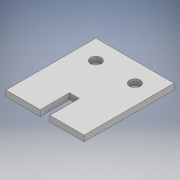
# Autodesk Inventor part: Camera_Mount
Saved by Autodesk Inventor 2017 (Build 210142000, 142)
## iProperties
Created: 2017-01-29
Part Number: Camera_Mount
Material: Generic
Document SubType Name: Modeling
Designer: willt
Density: 1 g/cm^3
Appearance: Default
Author: willt
Autodesk Inventor part; units mm, degrees
ref_plane "YZ Plane" through (0, 0, 0) normal (1, 0, 0) x (0, 1, 0)
ref_plane "XZ Plane" through (0, 0, 0) normal (0, 1, 0) x (-1, 0, 0)
ref_plane "XY Plane" through (0, 0, 0) normal (0, 0, 1) x (1, 0, 0)
sketch "Sketch1" plane through (0, 0, 0) normal (0, 0, 1) x (1, 0, 0)
  line L0 (0, 0) -> (40, 0)
  line L1 (40, 0) -> (40, 46)
  line L2 (40, 46) -> (0, 46)
  line L3 (0, 46) -> (0, 0)
  line L4 (20, 0) -> (20, 15) construction
  line L5 (20, 15) -> (22.5, 15)
  line L6 (22.5, 15) -> (22.5, 0)
  line L7 (20, 15) -> (17.5, 15)
  line L8 (17.5, 15) -> (17.5, 0)
  line L9 (0, 46) -> (0, 36) construction
  line L10 (0, 36) -> (10, 36) construction
  circle A0 centre (10, 36) radius 2.75
  line L11 (40, 36) -> (30, 36) construction
  circle A1 centre (30, 36) radius 2.75
  dimension "d0" = 40
  dimension "d1" = 46
  dimension "d2" = 15
  dimension "d3" = 2.5
  dimension "d4" = 2.5
  dimension "d5" = 10
  dimension "d6" = 10
  dimension "d7" = 5.5
  dimension "d8" = 10
  dimension "d9" = 5.5
  constraints: 24 end point, 5 perpendicular, 5 point on line, 2 centre point, 2 coincident, 2 horizontal, 2 parallel, 1 midpoint, 1 vertical
  measures "d0" distance of L2.end L1.end
  measures "d1" distance of L1.end L0.end
  measures "d2" distance of L4.start L4.end
  measures "d3" distance of L4.end L5.end
  measures "d4" distance of L4.end L7.end
  measures "d5" distance of L2.end L9.end
  measures "d6" distance of L9.end L10.end
  measures "d7" diameter of A0
  measures "d8" distance of L11.start L11.end
  measures "d9" diameter of A1
extrude "Extrusion1" add sketch "Sketch1" along normal blind 3 contours L3 L2 L1 L0 L6 L5 L7 L8
body "Solid1"
